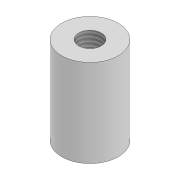
# Autodesk Inventor part: Tope para cerradura de leva
Saved by Autodesk Inventor 2020 (Build 240168000, 168)
## iProperties
Created: 2020-10-05
Part Number: Tope para cerradura de leva
Material: Genérico
Document SubType Name: Modeling
Designer: Pipi
Density: 1 g/cm^3
Appearance: Valor por defecto
Author: Pipi
Autodesk Inventor part; units mm, degrees
ref_plane "YZ Plane" through (0, 0, 0) normal (1, 0, 0) x (0, 1, 0)
ref_plane "XZ Plane" through (0, 0, 0) normal (0, 1, 0) x (-1, 0, 0)
ref_plane "XY Plane" through (0, 0, 0) normal (0, 0, 1) x (1, 0, 0)
sketch "Boceto1" plane through (0, 0, 0) normal (0, 1, 0) x (-1, 0, 0)
  circle A0 centre (0, 0) radius 5
  circle A1 centre (0, 0) radius 2
  dimension "d10" = 10
  dimension "d20" = 4
  constraints: 2 centre point, 1 coincident
  measures "d10" diameter of A0
  measures "d20" diameter of A1
extrude "Extrusión2" add sketch "Boceto1" along normal blind 15.5
thread "Thread1" size "M4x0.7" class "6H" standard "ISO Metric profile" length 15
